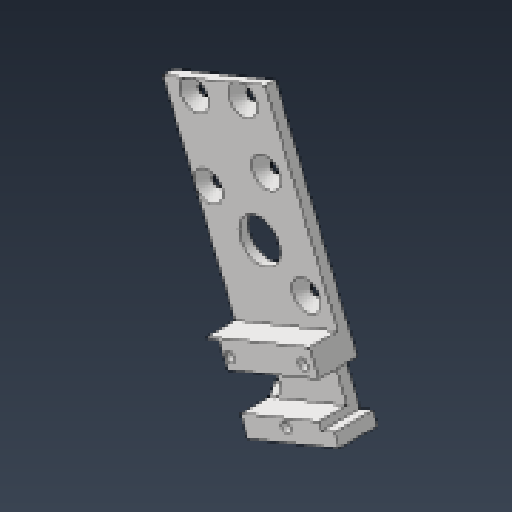
# Autodesk Inventor part: LeftGearboxCover
Saved by Autodesk Inventor 2026.2 (Build 302298010, 298A)
## iProperties
Created: 2026-04-04
Part Number: LeftGearboxCover
Material: Generic
Document SubType Name: Modeling
Designer: szymo
Density: 1 g/cm^3
Appearance: Default
Mass: 5.11258 g
Surface Area: 47.9452 cm^2
Volume: 5.11258 cm^3
Author: szymo
Autodesk Inventor part; units mm, degrees
ref_plane "YZ Plane" through (0, 0, 0) normal (1, 0, 0) x (0, 1, 0)
ref_plane "XZ Plane" through (0, 0, 0) normal (0, 1, 0) x (-1, 0, 0)
ref_plane "XY Plane" through (0, 0, 0) normal (0, 0, 1) x (1, 0, 0)
sketch "Sketch1" plane through (0, 0, 0) normal (0, 0, 1) x (1, 0, 0)
  circle A0 centre (0.0539, 16.4322) radius 13.85 construction
  circle A1 centre (0.0539, 16.4322) radius 14.5 construction
  circle A2 centre (15.5673, -21.2989) radius 13.85 construction
  circle A3 centre (15.5673, -21.2989) radius 14.5 construction
  circle A4 centre (-1.8632, 6.6177) radius 1.25 construction
  arc A5 (-1.5456, 14.6114) -> (-1.9501, 13.4922) centre (2.9234, 12.3633) ccw construction
  arc A6 (-1.9501, 13.4922) -> (-2.3098, 13.4782) centre (-1.8632, 6.6177) ccw construction
  arc A7 (-2.3098, 13.4782) -> (-2.8, 14.5627) centre (-7.0811, 11.9747) ccw construction
  arc A8 (-2.8, 14.5627) -> (-3.2145, 14.5028) centre (-1.8632, 6.6177) ccw construction
  arc A9 (-3.2145, 14.5028) -> (-3.3775, 13.3239) centre (1.6242, 13.2329) ccw construction
  arc A10 (-3.3775, 13.3239) -> (-3.7264, 13.2354) centre (-1.8632, 6.6177) ccw construction
  arc A11 (-3.7264, 13.2354) -> (-4.4314, 14.1943) centre (-8.0808, 10.7728) ccw construction
  arc A12 (-4.4314, 14.1943) -> (-4.8244, 14.0495) centre (-1.8632, 6.6177) ccw construction
  arc A13 (-4.8244, 14.0495) -> (-4.7387, 12.8625) centre (0.1726, 13.8134) ccw construction
  arc A14 (-4.7387, 12.8625) -> (-5.0616, 12.7034) centre (-1.8632, 6.6177) ccw construction
  arc A15 (-5.0616, 12.7034) -> (-5.9505, 13.4948) centre (-8.8088, 9.3893) ccw construction
  arc A16 (-5.9505, 13.4948) -> (-6.3048, 13.2714) centre (-1.8632, 6.6177) ccw construction
  arc A17 (-6.3048, 13.2714) -> (-5.9742, 12.1282) centre (-1.368, 14.0795) ccw construction
  arc A18 (-5.9742, 12.1282) -> (-6.257, 11.9055) centre (-1.8632, 6.6177) ccw construction
  arc A19 (-6.257, 11.9055) -> (-7.291, 12.4947) centre (-9.2333, 7.8846) ccw construction
  arc A20 (-7.291, 12.4947) -> (-7.5911, 12.2026) centre (-1.8632, 6.6177) ccw construction
  arc A21 (-7.5911, 12.2026) -> (-7.0301, 11.153) centre (-2.9302, 14.0194) ccw construction
  arc A22 (-7.0301, 11.153) -> (-7.2604, 10.8764) centre (-1.8632, 6.6177) ccw construction
  arc A23 (-7.2604, 10.8764) -> (-8.3943, 11.2378) centre (-9.3356, 6.3246) ccw construction
  arc A24 (-8.3943, 11.2378) -> (-8.6271, 10.8896) centre (-1.8632, 6.6177) ccw construction
  arc A25 (-8.6271, 10.8896) -> (-7.8601, 9.9796) centre (-4.4457, 13.6358) ccw construction
  arc A26 (-7.8601, 9.9796) -> (-8.0279, 9.6612) centre (-1.8632, 6.6177) ccw construction
  arc A27 (-8.0279, 9.6612) -> (-9.2121, 9.7789) centre (-9.1114, 4.7774) ccw construction
  arc A28 (-9.2121, 9.7789) -> (-9.3675, 9.39) centre (-1.8632, 6.6177) ccw construction
  arc A29 (-9.3675, 9.39) -> (-8.4281, 8.6594) centre (-5.8485, 12.9455) ccw construction
  arc A30 (-8.4281, 8.6594) -> (-8.5259, 8.313) centre (-1.8632, 6.6177) ccw construction
  arc A31 (-8.5259, 8.313) -> (-9.7088, 8.1819) centre (-8.5704, 3.3106) ccw construction
  arc A32 (-9.7088, 8.1819) -> (-9.7799, 7.7692) centre (-1.8632, 6.6177) ccw construction
  arc A33 (-9.7799, 7.7692) -> (-8.7091, 7.2498) centre (-7.077, 11.9786) ccw construction
  arc A34 (-8.7091, 7.2498) -> (-8.7328, 6.8907) centre (-1.8632, 6.6177) ccw construction
  arc A35 (-8.7328, 6.8907) -> (-9.8626, 6.5166) centre (-7.7362, 1.9884) ccw construction
  arc A36 (-9.8626, 6.5166) -> (-9.8463, 6.098) centre (-1.8632, 6.6177) ccw construction
  arc A37 (-9.8463, 6.098) -> (-8.6909, 5.8127) centre (-8.0777, 10.7775) ccw construction
  arc A38 (-8.6909, 5.8127) -> (-8.6394, 5.4564) centre (-1.8632, 6.6177) ccw construction
  arc A39 (-8.6394, 5.4564) -> (-9.6667, 4.8556) centre (-6.6454, 0.8685) ccw construction
  arc A40 (-9.6667, 4.8556) -> (-9.5638, 4.4496) centre (-1.8632, 6.6177) ccw construction
  arc A41 (-9.5638, 4.4496) -> (-8.3743, 4.4107) centre (-8.8067, 9.3945) ccw construction
  arc A42 (-8.3743, 4.4107) -> (-8.2499, 4.073) centre (-1.8632, 6.6177) ccw construction
  arc A43 (-8.2499, 4.073) -> (-9.1298, 3.2717) centre (-5.3456, -0.0002) ccw construction
  arc A44 (-9.1298, 3.2717) -> (-8.9448, 2.8959) centre (-1.8632, 6.6177) ccw construction
  arc A45 (-8.9448, 2.8959) -> (-7.7732, 3.1052) centre (-9.2323, 7.8902) ccw construction
  arc A46 (-7.7732, 3.1052) -> (-7.5813, 2.8007) centre (-1.8632, 6.6177) ccw construction
  arc A47 (-7.5813, 2.8007) -> (-8.2754, 1.834) centre (-3.8936, -0.5796) ccw construction
  arc A48 (-8.2754, 1.834) -> (-8.0162, 1.5049) centre (-1.8632, 6.6177) ccw construction
  arc A49 (-8.0162, 1.5049) -> (-6.9138, 1.9532) centre (-9.3359, 6.3303) ccw construction
  arc A50 (-6.9138, 1.9532) -> (-6.6627, 1.6953) centre (-1.8632, 6.6177) ccw construction
  arc A51 (-6.6627, 1.6953) -> (-7.1407, 0.6053) centre (-2.3528, -0.8444) ccw construction
  arc A52 (-7.1407, 0.6053) -> (-6.8188, 0.3374) centre (-1.8632, 6.6177) ccw construction
  arc A53 (-6.8188, 0.3374) -> (-5.8336, 1.0051) centre (-9.1128, 4.7829) ccw construction
  arc A54 (-5.8336, 1.0051) -> (-5.5344, 0.805) centre (-1.8632, 6.6177) ccw construction
  arc A55 (-5.5344, 0.805) -> (-5.7753, -0.3605) centre (-0.7906, -0.7831) ccw construction
  arc A56 (-5.7753, -0.3605) -> (-5.4047, -0.5557) centre (-1.8632, 6.6177) ccw construction
  arc A57 (-5.4047, -0.5557) -> (-4.5799, 0.3022) centre (-8.5729, 3.3157) ccw construction
  arc A58 (-4.5799, 0.3022) -> (-4.2456, 0.1687) centre (-1.8632, 6.6177) ccw construction
  arc A59 (-4.2456, 0.1687) -> (-4.2389, -1.0214) centre (0.7247, -0.3984) ccw construction
  arc A60 (-4.2389, -1.0214) -> (-3.8359, -1.1353) centre (-1.8632, 6.6177) ccw construction
  arc A61 (-3.8359, -1.1353) -> (-3.2075, -0.1246) centre (-7.7398, 1.9929) ccw construction
  arc A62 (-3.2075, -0.1246) -> (-2.8527, -0.1857) centre (-1.8632, 6.6177) ccw construction
  arc A63 (-2.8527, -0.1857) -> (-2.5988, -1.3484) centre (2.1268, 0.293) ccw construction
  arc A64 (-2.5988, -1.3484) -> (-2.1808, -1.376) centre (-1.8632, 6.6177) ccw construction
  arc A65 (-2.1808, -1.376) -> (-1.7763, -0.2567) centre (-6.6498, 0.8721) ccw construction
  arc A66 (-1.7763, -0.2567) -> (-1.4166, -0.2428) centre (-1.8632, 6.6177) ccw construction
  arc A67 (-1.4166, -0.2428) -> (-0.9264, -1.3273) centre (3.3546, 1.2607) ccw construction
  arc A68 (-0.9264, -1.3273) -> (-0.5119, -1.2673) centre (-1.8632, 6.6177) ccw construction
  arc A69 (-0.5119, -1.2673) -> (-0.3489, -0.0884) centre (-5.3506, 0.0025) ccw construction
  arc A70 (-0.3489, -0.0884) -> (0, 0) centre (-1.8632, 6.6177) ccw construction
  arc A71 (0, 0) -> (0.7049, -0.9589) centre (4.3544, 2.4627) ccw construction
  arc A72 (0.7049, -0.9589) -> (1.0979, -0.8141) centre (-1.8632, 6.6177) ccw construction
  arc A73 (1.0979, -0.8141) -> (1.0123, 0.3729) centre (-3.899, -0.578) ccw construction
  arc A74 (1.0123, 0.3729) -> (1.3352, 0.532) centre (-1.8632, 6.6177) ccw construction
  arc A75 (1.3352, 0.532) -> (2.2241, -0.2594) centre (5.0824, 3.8462) ccw construction
  arc A76 (2.2241, -0.2594) -> (2.5784, -0.036) centre (-1.8632, 6.6177) ccw construction
  arc A77 (2.5784, -0.036) -> (2.2478, 1.1073) centre (-2.3585, -0.844) ccw construction
  arc A78 (2.2478, 1.1073) -> (2.5306, 1.33) centre (-1.8632, 6.6177) ccw construction
  arc A79 (2.5306, 1.33) -> (3.5646, 0.7407) centre (5.5069, 5.3508) ccw construction
  arc A80 (3.5646, 0.7407) -> (3.8647, 1.0328) centre (-1.8632, 6.6177) ccw construction
  arc A81 (3.8647, 1.0328) -> (3.3037, 2.0824) centre (-0.7963, -0.784) ccw construction
  arc A82 (3.3037, 2.0824) -> (3.534, 2.359) centre (-1.8632, 6.6177) ccw construction
  arc A83 (3.534, 2.359) -> (4.6679, 1.9976) centre (5.6092, 6.9108) ccw construction
  arc A84 (4.6679, 1.9976) -> (4.9007, 2.3458) centre (-1.8632, 6.6177) ccw construction
  arc A85 (4.9007, 2.3458) -> (4.1337, 3.2558) centre (0.7193, -0.4004) ccw construction
  arc A86 (4.1337, 3.2558) -> (4.3014, 3.5742) centre (-1.8632, 6.6177) ccw construction
  arc A87 (4.3014, 3.5742) -> (5.4857, 3.4565) centre (5.385, 8.458) ccw construction
  arc A88 (5.4857, 3.4565) -> (5.6411, 3.8454) centre (-1.8632, 6.6177) ccw construction
  arc A89 (5.6411, 3.8454) -> (4.7016, 4.5761) centre (2.122, 0.2899) ccw construction
  arc A90 (4.7016, 4.5761) -> (4.7995, 4.9224) centre (-1.8632, 6.6177) ccw construction
  arc A91 (4.7995, 4.9224) -> (5.9824, 5.0535) centre (4.844, 9.9248) ccw construction
  arc A92 (5.9824, 5.0535) -> (6.0535, 5.4662) centre (-1.8632, 6.6177) ccw construction
  arc A93 (6.0535, 5.4662) -> (4.9827, 5.9856) centre (3.3506, 1.2568) ccw construction
  arc A94 (4.9827, 5.9856) -> (5.0064, 6.3447) centre (-1.8632, 6.6177) ccw construction
  arc A95 (5.0064, 6.3447) -> (6.1362, 6.7189) centre (4.0098, 11.247) ccw construction
  arc A96 (6.1362, 6.7189) -> (6.1199, 7.1374) centre (-1.8632, 6.6177) ccw construction
  arc A97 (6.1199, 7.1374) -> (4.9645, 7.4227) centre (4.3512, 2.4579) ccw construction
  arc A98 (4.9645, 7.4227) -> (4.913, 7.779) centre (-1.8632, 6.6177) ccw construction
  arc A99 (4.913, 7.779) -> (5.9403, 8.3798) centre (2.919, 12.3669) ccw construction
  arc A100 (5.9403, 8.3798) -> (5.8374, 8.7858) centre (-1.8632, 6.6177) ccw construction
  arc A101 (5.8374, 8.7858) -> (4.6479, 8.8247) centre (5.0803, 3.8409) ccw construction
  arc A102 (4.6479, 8.8247) -> (4.5235, 9.1625) centre (-1.8632, 6.6177) ccw construction
  arc A103 (4.5235, 9.1625) -> (5.4034, 9.9638) centre (1.6192, 13.2356) ccw construction
  arc A104 (5.4034, 9.9638) -> (5.2183, 10.3395) centre (-1.8632, 6.6177) ccw construction
  arc A105 (5.2183, 10.3395) -> (4.0468, 10.1302) centre (5.5059, 5.3452) ccw construction
  arc A106 (4.0468, 10.1302) -> (3.8548, 10.4347) centre (-1.8632, 6.6177) ccw construction
  arc A107 (3.8548, 10.4347) -> (4.549, 11.4015) centre (0.1671, 13.815) ccw construction
  arc A108 (4.549, 11.4015) -> (4.2898, 11.7305) centre (-1.8632, 6.6177) ccw construction
  arc A109 (4.2898, 11.7305) -> (3.1873, 11.2822) centre (5.6094, 6.9051) ccw construction
  arc A110 (3.1873, 11.2822) -> (2.9363, 11.5402) centre (-1.8632, 6.6177) ccw construction
  arc A111 (2.9363, 11.5402) -> (3.4142, 12.6301) centre (-1.3736, 14.0798) ccw construction
  arc A112 (3.4142, 12.6301) -> (3.0923, 12.898) centre (-1.8632, 6.6177) ccw construction
  arc A113 (3.0923, 12.898) -> (2.1072, 12.2304) centre (5.3864, 8.4525) ccw construction
  arc A114 (2.1072, 12.2304) -> (1.808, 12.4305) centre (-1.8632, 6.6177) ccw construction
  arc A115 (1.808, 12.4305) -> (2.0489, 13.5959) centre (-2.9358, 14.0186) ccw construction
  arc A116 (2.0489, 13.5959) -> (1.6783, 13.7911) centre (-1.8632, 6.6177) ccw construction
  arc A117 (1.6783, 13.7911) -> (0.8535, 12.9332) centre (4.8465, 9.9197) ccw construction
  arc A118 (0.8535, 12.9332) -> (0.5192, 13.0667) centre (-1.8632, 6.6177) ccw construction
  arc A119 (0.5192, 13.0667) -> (0.5125, 14.2568) centre (-4.4511, 13.6338) ccw construction
  arc A120 (0.5125, 14.2568) -> (0.1095, 14.3707) centre (-1.8632, 6.6177) ccw construction
  arc A121 (0.1095, 14.3707) -> (-0.519, 13.36) centre (4.0133, 11.2426) ccw construction
  arc A122 (-0.519, 13.36) -> (-0.8737, 13.4211) centre (-1.8632, 6.6177) ccw construction
  arc A123 (-0.8737, 13.4211) -> (-1.1277, 14.5838) centre (-5.8533, 12.9425) ccw construction
  arc A124 (-1.1277, 14.5838) -> (-1.5456, 14.6114) centre (-1.8632, 6.6177) ccw construction
  arc A125 (9.5083, 4.7273) -> (9.5495, 6.1549) centre (3.5709, 5.6133) ccw construction
  arc A126 (9.5495, 6.1549) -> (9.0708, 6.3081) centre (6.384, -2.9082) ccw construction
  arc A127 (9.0708, 6.3081) -> (8.2753, 5.1221) centre (13.6232, 2.395) ccw construction
  arc A128 (8.2753, 5.1221) -> (7.8525, 5.21) centre (6.384, -2.9082) ccw construction
  arc A129 (7.8525, 5.21) -> (7.596, 6.615) centre (1.8607, 4.8422) ccw construction
  arc A130 (7.596, 6.615) -> (7.0959, 6.6654) centre (6.384, -2.9082) ccw construction
  arc A131 (7.0959, 6.6654) -> (6.5644, 5.3398) centre (12.3624, 3.7842) ccw construction
  arc A132 (6.5644, 5.3398) -> (6.1325, 5.338) centre (6.384, -2.9082) ccw construction
  arc A133 (6.1325, 5.338) -> (5.5895, 6.6589) centre (0.3481, 3.7324) ccw construction
  arc A134 (5.5895, 6.6589) -> (5.0899, 6.6042) centre (6.384, -2.9082) ccw construction
  arc A135 (5.0899, 6.6042) -> (4.8456, 5.1971) centre (10.8403, 4.8809) ccw construction
  arc A136 (4.8456, 5.1971) -> (4.4235, 5.1055) centre (6.384, -2.9082) ccw construction
  arc A137 (4.4235, 5.1055) -> (3.6178, 6.2846) centre (-0.9006, 2.3323) ccw construction
  arc A138 (3.6178, 6.2846) -> (3.1405, 6.1272) centre (6.384, -2.9082) ccw construction
  arc A139 (3.1405, 6.1272) -> (3.194, 4.7001) centre (9.1235, 5.6372) ccw construction
  arc A140 (3.194, 4.7001) -> (2.8002, 4.5227) centre (6.384, -2.9082) ccw construction
  arc A141 (2.8002, 4.5227) -> (1.767, 5.5086) centre (-1.831, 0.7033) ccw construction
  arc A142 (1.767, 5.5086) -> (1.3328, 5.2554) centre (6.384, -2.9082) ccw construction
  arc A143 (1.3328, 5.2554) -> (1.6819, 3.8706) centre (7.2869, 6.02) ccw construction
  arc A144 (1.6819, 3.8706) -> (1.3336, 3.6152) centre (6.384, -2.9082) ccw construction
  arc A145 (1.3336, 3.6152) -> (0.1179, 4.3647) centre (-2.4023, -1.0837) ccw construction
  arc A146 (0.1179, 4.3647) -> (-0.2542, 4.0268) centre (6.384, -2.9082) ccw construction
  arc A147 (-0.2542, 4.0268) -> (0.3752, 2.7449) centre (5.4109, 6.0127) ccw construction
  arc A148 (0.3752, 2.7449) -> (0.0876, 2.4226) centre (6.384, -2.9082) ccw construction
  arc A149 (0.0876, 2.4226) -> (-1.2573, 2.903) centre (-2.5897, -2.9503) ccw construction
  arc A150 (-1.2573, 2.903) -> (-1.551, 2.4951) centre (6.384, -2.9082) ccw construction
  arc A151 (-1.551, 2.4951) -> (-0.6688, 1.372) centre (3.5774, 5.6154) ccw construction
  arc A152 (-0.6688, 1.372) -> (-0.8831, 0.997) centre (6.384, -2.9082) ccw construction
  arc A153 (-0.8831, 0.997) -> (-2.2985, 1.1873) centre (-2.3848, -4.8151) ccw construction
  arc A154 (-2.2985, 1.1873) -> (-2.501, 0.7273) centre (6.384, -2.9082) ccw construction
  arc A155 (-2.501, 0.7273) -> (-1.4046, -0.1879) centre (1.8666, 4.8456) ccw construction
  arc A156 (-1.4046, -0.1879) -> (-1.5363, -0.5992) centre (6.384, -2.9082) ccw construction
  arc A157 (-1.5363, -0.5992) -> (-2.9603, -0.7074) centre (-1.7967, -6.5966) ccw construction
  arc A158 (-2.9603, -0.7074) -> (-3.0627, -1.1995) centre (6.384, -2.9082) ccw construction
  arc A159 (-3.0627, -1.1995) -> (-1.8, -1.8667) centre (0.3532, 3.737) ccw construction
  arc A160 (-1.8, -1.8667) -> (-1.8433, -2.2964) centre (6.384, -2.9082) ccw construction
  arc A161 (-1.8433, -2.2964) -> (-3.2137, -2.6983) centre (-0.8511, -8.2169) ccw construction
  arc A162 (-3.2137, -2.6983) -> (-3.2115, -3.2009) centre (6.384, -2.9082) ccw construction
  arc A163 (-3.2115, -3.2009) -> (-1.8377, -3.591) centre (-0.8966, 2.3379) ccw construction
  arc A164 (-1.8377, -3.591) -> (-1.7907, -4.0203) centre (6.384, -2.9082) ccw construction
  arc A165 (-1.7907, -4.0203) -> (-3.0476, -4.6984) centre (0.4107, -9.6052) ccw construction
  arc A166 (-3.0476, -4.6984) -> (-2.941, -5.1895) centre (6.384, -2.9082) ccw construction
  arc A167 (-2.941, -5.1895) -> (-1.5161, -5.2854) centre (-1.8282, 0.7095) ccw construction
  arc A168 (-1.5161, -5.2854) -> (-1.3808, -5.6956) centre (6.384, -2.9082) ccw construction
  arc A169 (-1.3808, -5.6956) -> (-2.4693, -6.6202) centre (1.9336, -10.7007) ccw construction
  arc A170 (-2.4693, -6.6202) -> (-2.2629, -7.0784) centre (6.384, -2.9082) ccw construction
  arc A171 (-2.2629, -7.0784) -> (-0.8492, -6.876) centre (-2.401, -1.077) ccw construction
  arc A172 (-0.8492, -6.876) -> (-0.6316, -7.2491) centre (6.384, -2.9082) ccw construction
  arc A173 (-0.6316, -7.2491) -> (-1.5041, -8.3798) centre (3.651, -11.4557) ccw construction
  arc A174 (-1.5041, -8.3798) -> (-1.2069, -8.7851) centre (6.384, -2.9082) ccw construction
  arc A175 (-1.2069, -8.7851) -> (0.1338, -8.2932) centre (-2.5897, -2.9435) ccw construction
  arc A176 (0.1338, -8.2932) -> (0.4242, -8.6129) centre (6.384, -2.9082) ccw construction
  arc A177 (0.4242, -8.6129) -> (-0.1941, -9.9002) centre (5.4879, -11.8372) ccw construction
  arc A178 (-0.1941, -9.9002) -> (0.1809, -10.2349) centre (6.384, -2.9082) ccw construction
  arc A179 (0.1809, -10.2349) -> (1.39, -9.475) centre (-2.3863, -4.8085) ccw construction
  arc A180 (1.39, -9.475) -> (1.7405, -9.7273) centre (6.384, -2.9082) ccw construction
  arc A181 (1.7405, -9.7273) -> (1.4034, -11.1151) centre (7.3639, -11.8284) ccw construction
  arc A182 (1.4034, -11.1151) -> (1.8397, -11.3645) centre (6.384, -2.9082) ccw construction
  arc A183 (1.8397, -11.3645) -> (2.8644, -10.3698) centre (-1.7995, -6.5904) ccw construction
  arc A184 (2.8644, -10.3698) -> (3.2598, -10.5438) centre (6.384, -2.9082) ccw construction
  arc A185 (3.2598, -10.5438) -> (3.2185, -11.9713) centre (9.1971, -11.4297) ccw construction
  arc A186 (3.2185, -11.9713) -> (3.6972, -12.1246) centre (6.384, -2.9082) ccw construction
  arc A187 (3.6972, -12.1246) -> (4.4927, -10.9385) centre (-0.8551, -8.2114) ccw construction
  arc A188 (4.4927, -10.9385) -> (4.9156, -11.0265) centre (6.384, -2.9082) ccw construction
  arc A189 (4.9156, -11.0265) -> (5.172, -12.4314) centre (10.9073, -10.6586) ccw construction
  arc A190 (5.172, -12.4314) -> (5.6721, -12.4818) centre (6.384, -2.9082) ccw construction
  arc A191 (5.6721, -12.4818) -> (6.2036, -11.1562) centre (0.4056, -9.6006) ccw construction
  arc A192 (6.2036, -11.1562) -> (6.6355, -11.1544) centre (6.384, -2.9082) ccw construction
  arc A193 (6.6355, -11.1544) -> (7.1785, -12.4753) centre (12.4199, -9.5488) ccw construction
  arc A194 (7.1785, -12.4753) -> (7.6781, -12.4206) centre (6.384, -2.9082) ccw construction
  arc A195 (7.6781, -12.4206) -> (7.9224, -11.0135) centre (1.9277, -10.6973) ccw construction
  arc A196 (7.9224, -11.0135) -> (8.3445, -10.9219) centre (6.384, -2.9082) ccw construction
  arc A197 (8.3445, -10.9219) -> (9.1502, -12.101) centre (13.6686, -8.1488) ccw construction
  arc A198 (9.1502, -12.101) -> (9.6276, -11.9437) centre (6.384, -2.9082) ccw construction
  arc A199 (9.6276, -11.9437) -> (9.574, -10.5165) centre (3.6445, -11.4536) ccw construction
  arc A200 (9.574, -10.5165) -> (9.9678, -10.3392) centre (6.384, -2.9082) ccw construction
  arc A201 (9.9678, -10.3392) -> (11.0011, -11.325) centre (14.599, -6.5197) ccw construction
  arc A202 (11.0011, -11.325) -> (11.4353, -11.0719) centre (6.384, -2.9082) ccw construction
  arc A203 (11.4353, -11.0719) -> (11.0861, -9.687) centre (5.4811, -11.8365) ccw construction
  arc A204 (11.0861, -9.687) -> (11.4345, -9.4317) centre (6.384, -2.9082) ccw construction
  arc A205 (11.4345, -9.4317) -> (12.6501, -10.1812) centre (15.1704, -4.7328) ccw construction
  arc A206 (12.6501, -10.1812) -> (13.0222, -9.8432) centre (6.384, -2.9082) ccw construction
  arc A207 (13.0222, -9.8432) -> (12.3928, -8.5613) centre (7.3571, -11.8291) ccw construction
  arc A208 (12.3928, -8.5613) -> (12.6804, -8.2391) centre (6.384, -2.9082) ccw construction
  arc A209 (12.6804, -8.2391) -> (14.0253, -8.7194) centre (15.3577, -2.8661) ccw construction
  arc A210 (14.0253, -8.7194) -> (14.319, -8.3115) centre (6.384, -2.9082) ccw construction
  arc A211 (14.319, -8.3115) -> (13.4368, -7.1885) centre (9.1906, -11.4318) ccw construction
  arc A212 (13.4368, -7.1885) -> (13.6512, -6.8135) centre (6.384, -2.9082) ccw construction
  arc A213 (13.6512, -6.8135) -> (15.0666, -7.0037) centre (15.1529, -1.0013) ccw construction
  arc A214 (15.0666, -7.0037) -> (15.269, -6.5437) centre (6.384, -2.9082) ccw construction
  arc A215 (15.269, -6.5437) -> (14.1726, -5.6286) centre (10.9014, -10.6621) ccw construction
  arc A216 (14.1726, -5.6286) -> (14.3043, -5.2172) centre (6.384, -2.9082) ccw construction
  arc A217 (14.3043, -5.2172) -> (15.7283, -5.109) centre (14.5648, 0.7802) ccw construction
  arc A218 (15.7283, -5.109) -> (15.8307, -4.617) centre (6.384, -2.9082) ccw construction
  arc A219 (15.8307, -4.617) -> (14.568, -3.9498) centre (12.4148, -9.5534) ccw construction
  arc A220 (14.568, -3.9498) -> (14.6113, -3.52) centre (6.384, -2.9082) ccw construction
  arc A221 (14.6113, -3.52) -> (15.9817, -3.1181) centre (13.6191, 2.4005) ccw construction
  arc A222 (15.9817, -3.1181) -> (15.9796, -2.6155) centre (6.384, -2.9082) ccw construction
  arc A223 (15.9796, -2.6155) -> (14.6057, -2.2255) centre (13.6647, -8.1543) ccw construction
  arc A224 (14.6057, -2.2255) -> (14.5587, -1.7961) centre (6.384, -2.9082) ccw construction
  arc A225 (14.5587, -1.7961) -> (15.8156, -1.1181) centre (12.3573, 3.7887) ccw construction
  arc A226 (15.8156, -1.1181) -> (15.709, -0.6269) centre (6.384, -2.9082) ccw construction
  arc A227 (15.709, -0.6269) -> (14.2841, -0.531) centre (14.5963, -6.5259) ccw construction
  arc A228 (14.2841, -0.531) -> (14.1489, -0.1208) centre (6.384, -2.9082) ccw construction
  arc A229 (14.1489, -0.1208) -> (15.2373, 0.8038) centre (10.8344, 4.8843) ccw construction
  arc A230 (15.2373, 0.8038) -> (15.0309, 1.262) centre (6.384, -2.9082) ccw construction
  arc A231 (15.0309, 1.262) -> (13.6172, 1.0596) centre (15.169, -4.7394) ccw construction
  arc A232 (13.6172, 1.0596) -> (13.3996, 1.4327) centre (6.384, -2.9082) ccw construction
  arc A233 (13.3996, 1.4327) -> (14.2721, 2.5634) centre (9.117, 5.6393) ccw construction
  arc A234 (14.2721, 2.5634) -> (13.9749, 2.9687) centre (6.384, -2.9082) ccw construction
  arc A235 (13.9749, 2.9687) -> (12.6342, 2.4767) centre (15.3578, -2.8729) ccw construction
  arc A236 (12.6342, 2.4767) -> (12.3438, 2.7965) centre (6.384, -2.9082) ccw construction
  arc A237 (12.3438, 2.7965) -> (12.9621, 4.0838) centre (7.2802, 6.0207) ccw construction
  arc A238 (12.9621, 4.0838) -> (12.5872, 4.4185) centre (6.384, -2.9082) ccw construction
  arc A239 (12.5872, 4.4185) -> (11.378, 3.6585) centre (15.1543, -1.008) ccw construction
  arc A240 (11.378, 3.6585) -> (11.0275, 3.9109) centre (6.384, -2.9082) ccw construction
  arc A241 (11.0275, 3.9109) -> (11.3647, 5.2987) centre (5.4041, 6.0119) ccw construction
  arc A242 (11.3647, 5.2987) -> (10.9283, 5.5481) centre (6.384, -2.9082) ccw construction
  arc A243 (10.9283, 5.5481) -> (9.9036, 4.5534) centre (14.5676, 0.774) ccw construction
  arc A244 (9.9036, 4.5534) -> (9.5083, 4.7273) centre (6.384, -2.9082) ccw construction
  line L0 (8.8677, -39.1906) -> (2.7834, -24.3926) projected
  line L1 (9.7925, -38.8104) -> (8.8677, -39.1906) projected
  line L2 (3.7082, -24.0124) -> (9.7925, -38.8104) projected
  line L3 (3.7082, -24.0124) -> (2.7834, -24.3926) projected
  line L4 (3.3096, -26.9874) -> (2.1308, -24.1203) projected
  line L5 (2.1308, -24.1203) -> (3.5181, -23.5499) projected
  line L6 (3.5181, -23.5499) -> (3.1378, -22.625) projected
  line L7 (3.1378, -22.625) -> (0.8256, -23.5757) projected
  line L8 (0.8256, -23.5757) -> (2.3847, -27.3677) projected
  line L9 (2.3847, -27.3677) -> (3.3096, -26.9874) projected
  line L10 (8.4052, -39.3808) -> (7.4165, -36.9761) projected
  line L11 (7.4165, -36.9761) -> (6.4916, -37.3564) projected
  line L12 (6.4916, -37.3564) -> (7.6705, -40.2235) projected
  line L13 (7.6705, -40.2235) -> (9.9827, -39.2728) projected
  line L14 (9.9827, -39.2728) -> (9.7925, -38.8104) projected
  line L15 (9.7925, -38.8104) -> (8.4052, -39.3808) projected
  line L16 (7.6705, -40.2235) -> (32.6421, -29.9562)
  line L17 (32.6421, -29.9562) -> (7.8122, 30.4343)
  line L18 (7.8122, 30.4343) -> (-17.1595, 20.1671)
  line L19 (-17.1595, 20.1671) -> (7.6705, -40.2235)
  circle A245 centre (6.384, -2.9082) radius 9.6 construction
  circle A246 centre (6.384, -2.9082) radius 5.6 projected
  circle A247 centre (6.384, -2.9082) radius 5 projected
  line L20 (0.6355, -23.1133) -> (3.4101, -21.9725)
  line L21 (3.4101, -21.9725) -> (10.4451, -39.0827)
  line L22 (5.5016, -27.0593) -> (27.6986, -17.9328)
  line L23 (9.3043, -36.308) -> (31.5013, -27.1816)
  line L24 (28.3568, -28.4745) -> (15.16, 3.6223)
  circle A248 centre (23.8853, -16.7446) radius 0.75
  circle A249 centre (19.7785, -32.0015) radius 0.75
  point P0 (24.5541, -19.2258)
  point P1 (3.4101, -21.9725)
  dimension "d1" = 4.5
  dimension "d2" = 4.4
  dimension "d5" = 0.5
  dimension "d6" = 0.5
  dimension "d11" = 2
  dimension "d15" = 10
  dimension "d16" = 1
  dimension "d17" = 3
  dimension "d18" = 0
  dimension "d19" = 2.5491
  constraints: 18 end point, 7 perpendicular, 7 point on line, 2 centre point, 2 parallel, 1 coincident, 8 other
  measures "d1" distance edge to line of A1 L18
  measures "d5" distance between parallel lines of L20 L7
  measures "d6" distance between parallel lines of L21 L2
  measures "d11" distance edge to line of A3 L17
  measures "d15" distance between parallel lines of L22 L23
  measures "d17" distance between parallel lines of L16 L23
  measures "d18" distance from line of L23 A249.centre
  measures "d19" distance from line of L22 A248.centre
ref_plane "Work Plane4" through (-17.1595, -40.2235, -0.2) normal (0, 0, 1) x (0.9248762, 0.3802684, 0)
extrude "Extrusion1" add sketch "Sketch1" against normal up to surface (0.2 mm away) contours L21 L23 A249 L17 L16 | L21 L22 L24 L23 A249 | L21 L20 L19 L18 L17 L22 | A249 L23 | L23 A249 | A248 L24 | L24 A248
ref_plane "Work Plane7" through (-1.4059, -10.6981, 2.3) normal (0, 0, 1) x (0.9948859, 0.1010048, 0)
extrude "Extrusion2" add sketch "Sketch1" along normal up to surface (2.3 mm away) contours L21 L23 A249 L17 L16 | L21 L22 L24 L23 A249 | L21 L20 L19 L18 L17 L22 | A249 L23 | L23 A249 | A246 | A248 L24 | L24 A248
sketch "Sketch2" plane through (32.6421, -29.9562, -0.2) normal (0, 0, -1) x (-0.9248762, -0.3802684, 0)
  circle A0 centre (12.5, 55.2958) radius 1.15 projected
  circle A1 centre (12.5, 55.2958) radius 1.65
  circle A2 centre (18.0053, 46.9477) radius 1.25 projected
  point P0 (18.7985, 40.1186)
  dimension "d12" = 0.5
  constraints: 1 centre point
  measures "d12" radial gap between concentric circles of A0 A1
extrude "Extrusion3" cut sketch "Sketch2" against normal blind 2 contours A0 | A1
hole "Hole4" at (-1.8632, 6.6177, -0.2) direction (0, 0, 1) diameter 2.5 depth 2
sketch "Sketch4" plane through (7.6705, -40.2235, 2.3) normal (0, 0, 1) x (0.9248762, 0.3802684, 0)
  line L0 (23.6, 13) -> (23.6, 3) projected
  line L1 (2.9, 13) -> (23.6, 13)
  line L2 (27, 65.2958) -> (27, 13) projected
  line L3 (27, 18) -> (2.6484, 18)
  line L4 (2.9, 13) -> (2.9, 18)
  line L5 (2.9, 13) -> (2.9, 0)
  line L6 (27.4, 0) -> (3.4, 0)
  line L7 (2.9, 4.75) -> (23.6, 4.75)
  line L8 (27, 13) -> (23.6, 13) projected
  line L9 (23.6, 13) -> (27, 13)
  circle A0 centre (13, 35.0012) radius 5 projected
  line L10 (27, 13) -> (23.6, 13) projected
  line L11 (27, 65.2958) -> (27, 13) projected
  line L12 (0, 65.2958) -> (27, 65.2958) projected
  line L13 (0, 18.5) -> (0, 65.2958) projected
  line L14 (27, 0) -> (3, 0) projected
  line L15 (27, 3) -> (27, 0) projected
  line L16 (23.6, 3) -> (27, 3) projected
  line L17 (23.6, 13) -> (23.6, 3) projected
  line L18 (27, 19) -> (0, 19)
  line L19 (2.9, 18) -> (0, 18)
  line L20 (3, 18.5) -> (0, 18.5) projected
  line L21 (3, 0) -> (3, 18.5) projected
  circle A1 centre (14.325, 2.729) radius 0.75 projected
  circle A2 centre (23.925, 15.2781) radius 0.75 projected
  circle A3 centre (4.725, 15.2781) radius 0.75 projected
  line L22 (4.8832, 18.729) -> (23.7668, 18.729) projected
  arc A4 (23.7668, 18.729) -> (23.8056, 18.726) centre (23.825, 19.2256) ccw projected
  arc A5 (27.65, 14.729) -> (23.8056, 18.726) centre (23.65, 14.729) ccw projected
  line L23 (27.65, 4.729) -> (27.65, 14.729) projected
  arc A6 (22.65, -0.271) -> (27.65, 4.729) centre (22.65, 4.729) ccw projected
  line L24 (6, -0.271) -> (22.65, -0.271) projected
  arc A7 (1, 4.729) -> (6, -0.271) centre (6, 4.729) ccw projected
  line L25 (1, 14.729) -> (1, 4.729) projected
  arc A8 (4.8444, 18.726) -> (1, 14.729) centre (5, 14.729) ccw projected
  arc A9 (4.8444, 18.726) -> (4.8832, 18.729) centre (4.825, 19.2256) ccw projected
  line L26 (1.5, 0.229) -> (1.5, 16.229) projected
  line L27 (2.5, 0.229) -> (1.5, 0.229) projected
  line L28 (2.5, 16.229) -> (2.5, 0.229) projected
  line L29 (2.5, 16.229) -> (1.5, 16.229) projected
  point P0 (8.2015, 40.1186)
  point P1 (2.9, 0)
  point P2 (0, 0)
  point P3 (27, 0)
  point P4 (27, 19)
  point P5 (0, 19)
  point P6 (2.6484, 18)
  point P7 (3.4, 0)
  point P8 (2.5, 0)
  point P9 (3.4, 0)
  point P10 (27, 65.2958)
  point P11 (3, 4.75)
  point P12 (3, 0)
  point P13 (3, 18)
  point P14 (27, 18)
  point P15 (27, 19)
  point P16 (3, 13)
  point P17 (23.6, 4.75)
  point P18 (27, 13)
  constraints: 10 end point, 6 point on line, 2 perpendicular, 1 collinear, 1 horizontal, 1 parallel, 1 vertical, 15 other
ref_plane "Work Plane8" through (1.3703, -39.8432, 9.2) normal (0, 0, -1) x (-0.3802684, 0.9248762, 0)
extrude "Extrusion4" add sketch "Sketch4" along normal up to surface (6.9 mm away) contours L1 L21 L3 A5 L2 L8 | L0 L16 L15 A6 L6 A7 L21 L7 | L21 A8 A9 L22 A4 A5 L3 | A5 L3 L2 | A7 L6 L14 L21 | A5 A4 L22 A9 A8 L21 L20 L13 L18 L2 L3 | L15 L6 A6 | A1 | A2 | A3
sketch "Sketch5" plane through (27.6986, -17.9328, -0.2) normal (0, 0, -1) x (-0.9248762, -0.3802684, 0)
  circle A0 centre (12.675, -10) radius 0.75 projected
  circle A1 centre (3.075, 2.5491) radius 0.75 projected
  circle A2 centre (22.275, 2.5491) radius 0.75 projected
  line L0 (22.1168, 6) -> (3.2332, 6) projected
  arc A3 (3.1944, 5.997) -> (3.2332, 6) centre (3.175, 6.4966) ccw projected
  arc A4 (3.1944, 5.997) -> (-0.65, 2) centre (3.35, 2) ccw projected
  line L1 (-0.65, -8) -> (-0.65, 2) projected
  arc A5 (-0.65, -8) -> (4.35, -13) centre (4.35, -8) ccw projected
  line L2 (21, -13) -> (4.35, -13) projected
  arc A6 (21, -13) -> (26, -8) centre (21, -8) ccw projected
  line L3 (26, 2) -> (26, -8) projected
  arc A7 (26, 2) -> (22.1556, 5.997) centre (22, 2) ccw projected
  arc A8 (22.1168, 6) -> (22.1556, 5.997) centre (22.175, 6.4966) ccw projected
  point P0 (18.7985, 27.1186)
hole "Hole1" at (19.7785, -32.0015, -0.2) at (23.8853, -16.7446, -0.2) at (6.1277, -24.0457, -0.2) direction (0, 0, 1) diameter 3 depth 4.5 counterbore diameter 3.5 counterbore depth 0.5
hole "Hole3" at (19.7785, -32.0015, -0.2) at (6.1277, -24.0457, -0.2) at (23.8853, -16.7446, -0.2) direction (0, 0, 1) diameter 2.5 end through all
sketch "Sketch7" plane through (-17.1595, 20.1671, 2.3) normal (0, 0, 1) x (0.9248762, 0.3802684, 0)
  circle A0 centre (3.5, -3.2298) radius 2 projected
  circle A1 centre (3.5, -39.8863) radius 2.25 projected
  circle A2 centre (20.25, -43.7169) radius 2.25 projected
  circle A3 centre (19.75, -57.3419) radius 2.25 projected
  circle A4 centre (7, -57.3419) radius 2.25 projected
  circle A5 centre (21.258, -20.5803) radius 2.25 projected
  point P0 (8.2015, -25.1773)
hole "Hole5" at (-12.6942, 18.5109, 2.3) at (18.1934, -12.5652, 2.3) at (1.2451, -15.3919, 2.3) at (11.12, -30.2051, 2.3) at (22.9121, -25.3567, 2.3) at (10.3276, 9.2166, 2.3) direction (0, 0, -1) diameter 2.459 end through all countersink diameter 7 countersink angle 90 thread size "M3x0.5" class "6H" standard "ISO Metric profile"
equation "\"d6\" = d5"
body "Solid1"
